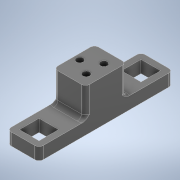
# Autodesk Inventor part: PotHolder
Saved by Autodesk Inventor 2022 (Build 260153000, 153)
## iProperties
Created: 2021-11-22
Part Number: PotHolder
Material: Genérico
Document SubType Name: Modeling
Designer: JK
Density: 1 g/cm^3
Appearance: Suave - Negro
Author: JK
Autodesk Inventor part; units mm, degrees
ref_plane "YZ Plane" through (0, 0, 0) normal (1, 0, 0) x (0, 1, 0)
ref_plane "XZ Plane" through (0, 0, 0) normal (0, 1, 0) x (-1, 0, 0)
ref_plane "XY Plane" through (0, 0, 0) normal (0, 0, 1) x (1, 0, 0)
sketch "Boceto7" plane through (0, 0, 0) normal (0, 1, 0) x (-1, 0, 0)
  line L0 (-7.8, 17.2) -> (7.8, 17.2)
  line L1 (7.8, 17.2) -> (7.8, -17.2)
  line L2 (7.8, -17.2) -> (-7.8, -17.2)
  line L3 (-7.8, -17.2) -> (-7.8, 17.2)
  line L4 (-7.8, 17.2) -> (7.8, -17.2) construction
  line L5 (7.8, 17.2) -> (-7.8, -17.2) construction
  line L6 (7.8, 17.2) -> (-7.8, 17.2)
  line L7 (-7.8, 17.2) -> (-7.8, 32.8)
  line L8 (-7.8, 32.8) -> (7.8, 32.8)
  line L9 (7.8, 32.8) -> (7.8, 17.2)
  line L10 (7.8, -17.2) -> (-7.8, -17.2)
  line L11 (-7.8, -17.2) -> (-7.8, -32.8)
  line L12 (-7.8, -32.8) -> (7.8, -32.8)
  line L13 (7.8, -32.8) -> (7.8, -17.2)
  line L14 (4.8, 29.8) -> (-4.8, 29.8)
  line L15 (-4.8, 29.8) -> (-4.8, 20.2)
  line L16 (-4.8, 20.2) -> (4.8, 20.2)
  line L17 (4.8, 20.2) -> (4.8, 29.8)
  line L18 (4.8, -20.2) -> (-4.8, -20.2)
  line L19 (-4.8, -20.2) -> (-4.8, -29.8)
  line L20 (-4.8, -29.8) -> (4.8, -29.8)
  line L21 (4.8, -29.8) -> (4.8, -20.2)
  line L22 (-4.8, 29.8) -> (4.8, 29.8)
  line L23 (4.8, 29.8) -> (4.8, 20.2)
  line L24 (4.8, 20.2) -> (-4.8, 20.2)
  line L25 (-4.8, 20.2) -> (-4.8, 29.8)
  line L26 (-4.8, 29.8) -> (4.8, 20.2) construction
  line L27 (4.8, 29.8) -> (-4.8, 20.2) construction
  line L28 (-4.8, -20.2) -> (4.8, -20.2)
  line L29 (4.8, -20.2) -> (4.8, -29.8)
  line L30 (4.8, -29.8) -> (-4.8, -29.8)
  line L31 (-4.8, -29.8) -> (-4.8, -20.2)
  line L32 (-4.8, -20.2) -> (4.8, -29.8) construction
  line L33 (4.8, -20.2) -> (-4.8, -29.8) construction
  point P0 (0, 0)
  point P1 (0, 25)
  point P2 (0, -25)
  dimension "d23" = 9.6
  dimension "d24" = 9.6
  dimension "d25" = 3
  dimension "d26" = 3
  dimension "d27" = 3
  dimension "d28" = 3
  dimension "d29" = 3
  dimension "d30" = 3
  dimension "d31" = 3
  dimension "d43" = 50
  constraints: 68 end point, 14 parallel, 7 horizontal, 7 perpendicular, 6 midpoint, 5 collinear, 2 equal length, 1 point on line
  measures "d23" distance of L16.end L14.start
  measures "d24" distance of L15.end L16.end
  measures "d25" distance between parallel lines of L9 L17
  measures "d26" distance between parallel lines of L14 L8
  measures "d27" distance between parallel lines of L7 L15
  measures "d28" distance between parallel lines of L0 L16
  measures "d29" distance between parallel lines of L11 L19
  measures "d30" distance between parallel lines of L12 L20
  measures "d31" distance between parallel lines of L2 L18
  measures "d43" distance of point (0, -25) point (0, 25)
extrude "Extrusión4" add sketch "Boceto7" along normal blind 6
sketch "Boceto8" plane through (0, 6, 0) normal (0, 1, 0) x (1, 0, 0)
  circle A0 centre (-5, 0) radius 1.7
  point P0 (0, 0)
  dimension "d35" = 3.4
  dimension "d36" = 5
  constraints: 1 centre point, 1 horizontal alignment
  measures "d35" diameter of A0
  measures "d36" distance of point (0, 0) A0.centre
extrude "Extrusión5" cut sketch "Boceto8" against normal through all
pattern_circular "Patrón circular1" count 3 over 360 about axis through (0, -10, 0) along (0, 1, 0) of "Extrusión5"
fillet "Empalme3" radius 2 4 edges at (-7.8, 3, 32.8) (7.8, 3, 32.8) (-7.8, 3, -32.8) (7.8, 3, -32.8)
sketch "Boceto9" plane through (0, 6, 0) normal (0, 1, 0) x (1, 0, 0)
  line L0 (-7.8, 30.8) -> (-7.8, -30.8) projected
  line L1 (7.8, -10) -> (-7.8, -10)
  line L2 (-7.8, -10) -> (-7.8, 10)
  line L3 (-7.8, 10) -> (7.8, 10)
  line L4 (7.8, 10) -> (7.8, -10)
  line L5 (7.8, -10) -> (-7.8, 10) construction
  line L6 (-7.8, -10) -> (7.8, 10) construction
  arc A0 (7.8, 30.8) -> (5.8, 32.8) centre (5.8, 30.8) ccw projected
  line L7 (5.8, 32.8) -> (-5.8, 32.8) projected
  arc A1 (-5.8, 32.8) -> (-7.8, 30.8) centre (-5.8, 30.8) ccw projected
  line L8 (-7.8, 30.8) -> (-7.8, -30.8) projected
  arc A2 (-7.8, -30.8) -> (-5.8, -32.8) centre (-5.8, -30.8) ccw projected
  line L9 (-5.8, -32.8) -> (5.8, -32.8) projected
  arc A3 (5.8, -32.8) -> (7.8, -30.8) centre (5.8, -30.8) ccw projected
  line L10 (7.8, -30.8) -> (7.8, 30.8) projected
  circle A4 centre (2.5, 4.3301) radius 1.7 projected
  circle A5 centre (2.5, -4.3301) radius 1.7 projected
  circle A6 centre (-5, 0) radius 1.7 projected
  line L11 (-4.8, -29.8) -> (-4.8, -20.2) projected
  line L12 (-4.8, -20.2) -> (4.8, -20.2) projected
  line L13 (4.8, -20.2) -> (4.8, -29.8) projected
  line L14 (4.8, -29.8) -> (-4.8, -29.8) projected
  line L15 (-4.8, 20.2) -> (-4.8, 29.8) projected
  line L16 (-4.8, 29.8) -> (4.8, 29.8) projected
  line L17 (4.8, 29.8) -> (4.8, 20.2) projected
  line L18 (4.8, 20.2) -> (-4.8, 20.2) projected
  point P0 (0, 0)
  dimension "d44" = 20
  constraints: 12 end point, 2 midpoint, 2 parallel, 1 horizontal, 1 perpendicular, 1 point on line
  measures "d44" distance between parallel lines of L3 L1
extrude "Extrusión6" add sketch "Boceto9" along normal blind 14.6 contours L3 L4 L1 L0
fillet "Empalme4" radius 2 6 edges at (7.8, 13.3, 10) (7.8, 13.3, -10) (-7.8, 13.3, -10) (-7.8, 13.3, 10) (0, 6, -10) (0, 6, 10)
